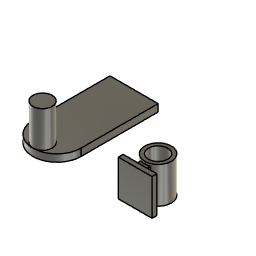
move-detector-bottom-holder v3 (Autodesk Fusion 360 design; units mm, degrees)
Autodesk Fusion 360 part; units mm, degrees
box "BoxPrimitive1" add length 30 width 20 height 3 placed x (0, 1, 0) y (-1, 0, 0) z (0, 0, 1) at (20, 0, 0) makes body 1
extrude "Extrude1" add 1 faces at (13.3333, 0, 1) along direction (0, -1, 0) blind 10 on bodies 1 bodies 1
extrude "Extrude2" add 1 faces at (13.3333, -10, 1) along direction (0, -1, 0) blind 2 on bodies 1 bodies 1
cylinder "CylinderPrimitive1" add diameter 8 height 20 placed x (1, 0, 0) y (0, 1, 0) z (0, 0, 1) at (10, -8, 3) bodies 1
fillet "Fillet1" radius 10 2 edges at (20, -12, 1.5) (0, -12, 1.5) on bodies 1
extrude "Extrude3" cut 1 faces at (10.435, -8.7534, 23) along direction (0, 0, -1) blind 5 on bodies 1 bodies 1
cylinder "CylinderPrimitive2" add diameter 11 height 12 placed x (1, 0, 0) y (0, 1, 0) z (0, 0, 1) at (50, 0, 0) separate body makes body 2
hole "Hole1" at (50, 0, 12) direction (0, 0, -1) diameter 8.5 depth 15 tip angle 180 bodies 2
hole "Hole2" at (55.5, 0, 6) direction (-1, 0, 0) diameter 3 depth 5 tip angle 180 bodies 2
cylinder "CylinderPrimitive3" add diameter 4 height 2 placed x (1, 0, 0) y (0, 0, -1) z (0, 1, 0) at (50, 0, 6) separate body makes body 3
move_body "Move1" bodies 3 to x (1, 0, 0) y (0, 1, 0) z (0, 0, 1) at (0, -7.5, 0)
extrude "Extrude4" add 1 faces at (49.9118, -5.5, 5.5033) along direction (0, 1, 0) blind 1 on bodies 3 bodies 2 3
box "BoxPrimitive2" add length 9 width 8 height 2 placed x (0, 0, -1) y (1, 0, 0) z (0, -1, 0) at (46, -7.5, 9) bodies 2
box "BoxPrimitive3" add length 2.5 width 4 height -8 placed x (0, 1, 0) y (1, 0, 0) z (0, 0, -1) at (48, -7.5, 0) bodies 2
extrude "Extrude5" add 1 faces at (54, -8.1667, 6) along direction (1, 0, 0) blind 3 on bodies 2 bodies 2
extrude "Extrude6" add 1 faces at (46, -8.1667, 6) along direction (-1, 0, 0) blind 3 on bodies 2 bodies 2
extrude "Extrude7" add 1 faces at (55.0589, -0.3791, 12) along direction (0, 0, 1) blind 3 on bodies 2 bodies 2
extrude "Extrude8" add 1 faces at (52.3333, -8.1667, 9) along direction (0, 0, 1) blind 6 on bodies 2 bodies 2
extrude "Extrude9" add 1 faces at (50.1363, -6.8283, 8) along direction (0, 0, 1) blind 6 on bodies 2 bodies 2
extrude "Extrude10" add 1 faces at (55.0589, -0.3791, 15) along direction (0, 0, -1) blind 12 on bodies 2 bodies 2
sketch "Sketch7" plane through (0, 0, 15) normal (0, 0, 1) x (-1, 0, 0)
  circle A0 centre (-50, 0) radius 4.25
  circle A1 centre (-50, 0) radius 5.5
  circle A2 centre (-50, 0) radius 4
  dimension "d51" = 8
  constraint concentric A0 A2
  measures "d51" diameter of A2
extrude "Extrude11" add sketch "Sketch7" against normal blind 15 contours A0 bodies 2
hole "Hole3" at (44.5, 0, 8) direction (1, 0, 0) diameter 2 depth 5 tip angle 180 bodies 2
